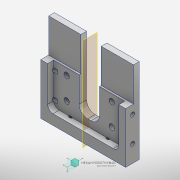
# Autodesk Inventor part: Z-head-beltmount
Saved by Autodesk Inventor 2016 (Build 200138000, 138)
## iProperties
Created: 2015-05-16
Part Number: Z-head-beltmount
Material: Aluminum 6061
Document SubType Name: Modeling
Designer: as
Mass: 25.7765 g
Surface Area: 63.5364 cm^2
Volume: 9.54684 cm^3
Density: 2.7 g/cm^3
Appearance: Aluminum - Flat
Author: as
Autodesk Inventor part; units mm, degrees
ref_plane "YZ Plane" through (0, 0, 0) normal (1, 0, 0) x (0, 1, 0)
ref_plane "XZ Plane" through (0, 0, 0) normal (0, 1, 0) x (-1, 0, 0)
ref_plane "XY Plane" through (0, 0, 0) normal (0, 0, 1) x (1, 0, 0)
sketch "Sketch1" plane through (0, 0, 0) normal (0, 0, 1) x (1, 0, 0)
  line L0 (15.16, -27.5645) -> (-34.84, -27.5645)
  line L1 (-34.84, -27.5645) -> (-34.84, -19.5645)
  line L2 (-34.84, -19.5645) -> (15.16, -19.5645)
  line L3 (15.16, -19.5645) -> (15.16, -27.5645)
  point P0 (0, 0)
  dimension "d0" = 50
  dimension "d1" = 8
  constraints: 8 end point, 2 parallel, 1 horizontal, 1 perpendicular
  measures "d0" distance of L1.end L2.end
  measures "d1" distance of L0.end L1.end
extrude "Extrusion1" add sketch "Sketch1" along normal blind 50
sketch "Sketch3" plane through (-34.84, -27.5645, 0) normal (0, -1, 0) x (1, 0, 0)
  line L0 (0, 50) -> (50, 50) projected
  line L1 (0, 50) -> (50, 50)
  line L2 (50, 50) -> (50, 30)
  line L3 (50, 30) -> (0, 30)
  line L4 (0, 30) -> (0, 50)
  point P0 (34.84, 0)
  dimension "d8" = 50
  dimension "d9" = 20
  constraints: 8 end point, 2 parallel, 1 horizontal, 1 perpendicular
  measures "d8" distance of L2.end L3.end
  measures "d9" distance of L1.end L2.end
extrude "Extrusion3" cut sketch "Sketch3" against normal blind 4.66
sketch "Sketch4" plane through (-34.84, -27.5645, 0) normal (0, -1, 0) x (1, 0, 0)
  line L0 (50, 30) -> (0, 30) projected
  line L1 (46, 30) -> (4, 30)
  line L2 (4, 30) -> (4, 9.2)
  line L3 (7.2, 6) -> (42.8, 6)
  line L4 (46, 9.2) -> (46, 30)
  line L5 (50, 0) -> (50, 30) projected
  line L6 (0, 0) -> (0, 30) projected
  line L7 (50, 0) -> (0, 0) projected
  arc A0 (42.8, 6) -> (46, 9.2) centre (42.8, 9.2) ccw
  arc A1 (4, 9.2) -> (7.2, 6) centre (7.2, 9.2) ccw
  point P0 (34.84, 0)
  dimension "d12" = 4
  dimension "d13" = 4
  dimension "d14" = 6
  dimension "d15" = 3.2
  constraints: 8 end point, 4 point on circle, 4 tangent, 2 centre point, 2 parallel, 1 equal radius, 1 horizontal, 1 perpendicular, 1 point on line
  measures "d12" distance between parallel lines of L5 L4
  measures "d13" distance between parallel lines of L6 L2
  measures "d14" distance between parallel lines of L7 L3
  measures "d15" radius of A0
extrude "Extrusion4" cut sketch "Sketch4" against normal blind 3.6 contours L4 A0 L3 A1 L2 L0
sketch "Sketch2" plane through (-34.84, -27.5645, 0) normal (0, -1, 0) x (1, 0, 0)
  line L0 (31, 15) -> (31, 50)
  line L1 (31, 50) -> (19, 50)
  line L2 (19, 50) -> (19, 15)
  line L3 (24, 10) -> (26, 10)
  line L4 (31, 10) -> (19, 50) construction
  line L5 (31, 50) -> (19, 10) construction
  arc A0 (26, 10) -> (31, 15) centre (26, 15) ccw
  arc A1 (19, 15) -> (24, 10) centre (24, 15) ccw
  line L6 (0, 0) -> (0, 30) projected
  line L7 (50, 0) -> (0, 0) projected
  point P0 (34.84, 0)
  point P1 (25, 30)
  dimension "d4" = 12
  dimension "d5" = 5
  dimension "d18" = 25
  dimension "d20" = 50
  dimension "d21" = 10
  constraints: 12 end point, 4 point on circle, 4 point on line, 4 tangent, 3 parallel, 2 centre point, 2 midpoint, 1 equal radius, 1 perpendicular
  measures "d4" distance of L1.end L0.end
  measures "d5" radius of A0
  measures "d18" distance from line of L6 point (25, 30)
  measures "d20" distance from line of point (34.84, 0) L1
  measures "d21" distance between parallel lines of L7 L3
extrude "Extrusion2" cut sketch "Sketch2" against normal through all
hole "Hole1" at (15.16, -23.5645, 10) direction (-1, 0, 0) diameter 2.459 depth 6 tip angle 118 thread size "M3x0.5" class "6H" standard "ISO Metric profile"
pattern_linear "Rectangular Pattern1" count 2 spacing 15 along (0, 0, 1) of "Hole1"
hole "Hole2" at (11.16, -23.5645, 0) direction (0, 0, 1) diameter 2.459 depth 6 tip angle 118 thread size "M3x0.5" class "6H" standard "ISO Metric profile"
pattern_linear "Rectangular Pattern2" count 2 spacing 10 along (-1, 0, 0) of "Hole2"
ref_plane "Work Plane1" through (-9.84, -27.5645, 0) normal (1, 0, 0) x (0, 0, -1)
mirror "Mirror1" about plane through (-9.84, -27.5645, 0) normal (1, 0, 0) of "Hole1", "Rectangular Pattern1", "Hole2", "Rectangular Pattern2"
sketch "Sketch5" plane through (0, 0, 0) normal (0, 0, -1) x (-1, 0, 0)
  point P0 (20.84, -23.5645)
sketch "Sketch6" plane through (-34.84, -27.5645, 0) normal (-1, 0, 0) x (0, 0, 1)
  point P0 (25, 4)
  point P1 (10, 4)
sketch "Sketch7" plane through (-34.84, -23.9645, 0) normal (0, -1, 0) x (1, 0, 0)
  point P0 (11.6661, 26)
  point P1 (11.6661, 13)
hole "Hole7" at (-23.1739, -23.9645, 26) at (-23.1739, -23.9645, 13) direction (0, 1, 0) diameter 3.242 depth 6 tip angle 120 thread size "M4x0.7" class "6H" standard "ISO Metric profile"
mirror "Mirror2" about plane through (-9.84, -27.5645, 0) normal (1, 0, 0) of "Hole7"
equation "\"d8\" = d0"
equation "\"d13\" = d12"
body "Solid1"
